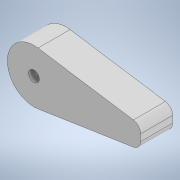
# Autodesk Inventor part: o_Plattenstopper
Saved by Autodesk Inventor 2020.3 (Build 243373000, 373)
## iProperties
Created: 2020-10-07
Part Number: o_Plattenstopper
Material: Generic
Document SubType Name: Modeling
Designer: Mara
Density: 1 g/cm^3
Appearance: Default
Author: Mara
Autodesk Inventor part; units mm, degrees
ref_plane "YZ Plane" through (0, 0, 0) normal (1, 0, 0) x (0, 1, 0)
ref_plane "XZ Plane" through (0, 0, 0) normal (0, 1, 0) x (-1, 0, 0)
ref_plane "XY Plane" through (0, 0, 0) normal (0, 0, 1) x (1, 0, 0)
sketch "Sketch1" plane through (0, 0, 0) normal (0, 0, 1) x (1, 0, 0)
  circle A0 centre (0, 0) radius 12.5
  line L0 (0, 0) -> (50, 0) construction
  line L1 (1.8894, 12.3564) -> (50, 5)
  line L2 (1.8894, -12.3564) -> (50, -5)
  line L3 (50, 5) -> (50, -5)
  dimension "d0" = 25
  dimension "d1" = 50
  dimension "d2" = 5
  dimension "d3" = 5
  dimension "d4" = 50
  constraints: 8 end point, 2 point on circle, 2 tangent, 1 centre point, 1 coincident, 1 horizontal, 1 vertical
  measures "d0" diameter of A0
  measures "d1" distance of L0.start L0.end
  measures "d2" distance of L0.end L1.end
  measures "d3" distance of L0.end L2.end
  measures "d4" distance from line of point (0, 0) L3
extrude "Extrusion1" add sketch "Sketch1" along normal blind 15
fillet "Fillet1" radius 4 2 edges at (50, 5, 7.5) (50, -5, 7.5)
sketch "Sketch2" plane through (0, 0, 15) normal (0, 0, 1) x (1, 0, 0)
  circle A0 centre (0, 0) radius 2.5
  dimension "d8" = 5
  constraints: 1 centre point, 1 coincident
  measures "d8" diameter of A0
extrude "Extrusion2" cut sketch "Sketch2" against normal through all
equation "\"d4\" = d1"
body "Solid1"
